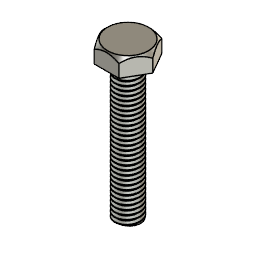
smartie_hopper (Autodesk Fusion 360 archive; units mm, degrees)
design "M6 32 mm Hex Bolt"
part number: 2026-04-25-09-17-42-437
Autodesk Fusion 360 part; units mm, degrees
sketch "Thread" plane through (0, 0, 0) normal (0, 0, 1) x (1, 0, 0)
  circle A0 centre (0, 0) radius 3
  dimension "d2" = 6
  constraint coincident A0.centre origin
  measures "d2" diameter of A0
extrude "Extrude1" add sketch "Thread" along normal blind 32
sketch "Head" plane through (0, 0, 32) normal (0, 0, 1) x (-1, 0, 0)
  circle A0 centre (0, 0) radius 3
  line L0 (2.8868, -5) -> (5.7735, 0)
  line L1 (5.7735, 0) -> (2.8868, 5)
  line L2 (2.8868, 5) -> (-2.8868, 5)
  line L3 (-2.8868, 5) -> (-5.7735, 0)
  line L4 (-5.7735, 0) -> (-2.8868, -5)
  line L5 (-2.8868, -5) -> (2.8868, -5)
  dimension "d10" = 10
  constraint coincident A0.centre origin
  measures "d10" distance of L2 L5
extrude "Extrude2" add sketch "Head" along normal blind 4 contours A0 | L0 L1 L2 L3 L4 L5
thread "Thread1" "ISO Metric profile 6.0 M6x1 M6x1 6g" major diameter 5.884 minor diameter 4.7435 pitch 1 angle 60 modelled right hand crest width 0.1444 on face at (2.9963, -0.1495, 21.3333) crest through (2.942, 0, -0.25)
sketch "Head fillet" plane through (0, 0, 0) normal (0, 1, 0) x (1, 0, 0)
  line L0 (2.8868, -32) -> (5.7735, -32)
  line L1 (5.7735, -32) -> (5.7735, -36)
  line L2 (5.7735, -36) -> (2.8868, -36)
  line L3 (2.8868, -36) -> (2.8868, -32)
  line L4 (-5.7735, -32) -> (-2.8868, -32)
  line L5 (-2.8868, -32) -> (-2.8868, -36)
  line L6 (-2.8868, -36) -> (-5.7735, -36)
  line L7 (-5.7735, -36) -> (-5.7735, -32)
  line L8 (-2.8868, -32) -> (2.8868, -32)
  line L9 (2.8868, -32) -> (2.8868, -36)
  line L10 (2.8868, -36) -> (-2.8868, -36)
  line L11 (-2.8868, -36) -> (-2.8868, -32)
  line L12 (5.7735, -36) -> (4.7735, -36)
  line L13 (5.7735, -36) -> (5.7735, -35)
  line L14 (4.7735, -36) -> (5.7735, -35)
  dimension "d14" = 1
  dimension "d15" = 1
  constraint coincident L1.end L2.start
  constraint perpendicular L1 L12
  constraint perpendicular L2 L13
  measures "d14" distance of L1.end L12.end
  measures "d15" distance of L1.end L13.end
revolve "Revolve1" cut sketch "Head fillet" angle 360 about axis through (0, 0, 1.75) along (0, 0, 1) contours L1 L2 L12 L13 L14
equation "diameter = 6 mm" comment "An M6 hex bolt has a diameter of 6 mm."
equation "d2 = diameter"
equation "thread_height = 32 mm" comment "The length of the M6 hex bolt (excluding the head)."
equation "d4 = thread_height"
equation "head_height = 4 mm" comment "An M6 hex bolt has a head thickness of 4 mm."
equation "width_across_flats = 10 mm" comment "An M6 hex bolt has a width across the flats of 10 mm."
equation "d10 = width_across_flats"
equation "d11 = head_height"
equation "chamfer_side_length = 1 mm" comment "Chamfer on the top of the hex bolt head."
equation "d14 = chamfer_side_length"
equation "d15 = chamfer_side_length"
named bodies: "M6 32 mm Hex Bolt"

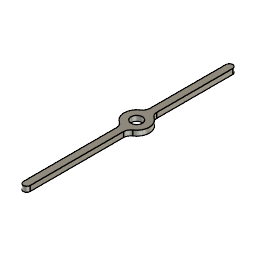
design "Mixer Arm"
part number: 2026-05-20-12-12-58-237
Autodesk Fusion 360 part; units mm, degrees
sketch "Mixer arm" plane through (0, 0, 0) normal (0, 0, 1) x (1, 0, 0)
  circle A0 centre (0, 0) radius 7.25
  circle A1 centre (0, 0) radius 3.25
  line L0 (-2, 55.25) -> (2, 55.25)
  line L1 (2, 55.25) -> (2, 3.25)
  line L2 (2, 3.25) -> (-2, 3.25)
  line L3 (-2, 3.25) -> (-2, 55.25)
  line L4 (-2, -3.25) -> (2, -3.25)
  line L5 (2, -3.25) -> (2, -65.25)
  line L6 (2, -65.25) -> (-2, -65.25)
  line L7 (-2, -65.25) -> (-2, -3.25)
  line L8 (-2, -7.25) -> (2, -7.25)
  line L9 (-2, 7.25) -> (2, 7.25)
  dimension "d3" = 6.5
  dimension "d5" = 14.5
  dimension "d6" = 2
  dimension "d7" = 2
  dimension "d8" = 2
  dimension "d9" = 2
  dimension "d14" = 58
  dimension "d15" = 48
  constraint coincident A0.centre A1.centre
  constraint concentric A0 A1
  constraint horizontal L0
  constraint vertical L1
  constraint horizontal L2
  constraint vertical L3
  constraint horizontal L4
  constraint vertical L5
  constraint horizontal L6
  constraint vertical L7
  constraint tangent A1 L2
  constraint tangent A1 L4
  constraint coincident L7 L8.start
  constraint coincident L5 L8.end
  constraint perpendicular L5 L8
  constraint tangent A0 L8
  constraint coincident L1 L9.end
  constraint perpendicular L1 L9
  constraint tangent A0 L9
  measures "d3" diameter of A1
  measures "d5" diameter of A0
  measures "d6" distance of A0.centre L1
  measures "d7" distance of A0.centre L3
  measures "d8" distance of A0.centre L7
  measures "d9" distance of A0.centre L5
  measures "d14" distance of L6 L8
  measures "d15" distance of L0 L9
extrude "Extrude1" add sketch "Mixer arm" along normal blind 3 contours A0 A1 L1 L2 L4 L5 | A0 L1 L2 L3 | A0 L1 L9 | A0 L5 L8 | A0 L4 L5 L7 | A0 L3 L9 | L0 L1 L3 L9 | A0 L7 L8 | L5 L6 L7 L8 | A0 A1 L2 L3 L4 L7
fillet "Fillet1" radius 4 4 edges at (2, -6.9687, 1.5) (2, 6.9687, 1.5) (-2, 6.9687, 1.5) (-2, -6.9687, 1.5)
fillet "Fillet2" radius 2 4 edges at (2, 55.25, 1.5) (-2, 55.25, 1.5) (-2, -65.25, 1.5) (2, -65.25, 1.5)
equation "stainless_steel_thickness = 3 mm" comment "The thickness of the 316 stainless steel sheets to laser cut."
equation "hole_diameter = 6.5 mm"
equation "d3 = hole_diameter"
equation "arm_thickness = 4 mm"
equation "d5 = hole_diameter + 2 * arm_thickness"
equation "d6 = arm_thickness / 2"
equation "d7 = arm_thickness / 2"
equation "d8 = arm_thickness / 2"
equation "d9 = arm_thickness / 2"
equation "d10 = stainless_steel_thickness"
equation "arm_length_front = 58 mm"
equation "arm_length_back = 48 mm"
equation "d14 = arm_length_front"
equation "d15 = arm_length_back"
equation "d17 = arm_thickness"
equation "d19 = arm_thickness / 2"
named bodies: "Mixer arm"

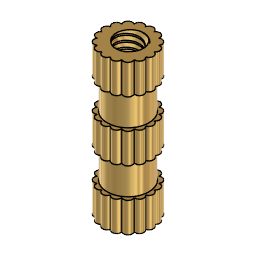
design "M2 10 mm Threaded Brass Insert"
part number: 2026-06-20-09-24-02-047
Autodesk Fusion 360 part; units mm, degrees
sketch "Brass thread outline" plane through (0, 0, 0) normal (0, 0, 1) x (1, 0, 0)
  circle A0 centre (0, 0) radius 1.4
  dimension "d4" = 2.8
  constraint coincident A0.centre origin
  measures "d4" diameter of A0
extrude "Extrude1" add sketch "Brass thread outline" along normal blind 10
sketch "Ridges" plane through (0, 0, 10) normal (0, 0, 1) x (-1, 0, 0)
  circle A0 centre (0, 0) radius 1.4
  circle A1 centre (0, 0) radius 1.7
  circle A2 centre (-0.0001, -1.4) radius 0.3
  circle A3 centre (0.5357, -1.2935) radius 0.3
  circle A4 centre (0.9899, -0.99) radius 0.3
  circle A5 centre (1.2934, -0.5358) radius 0.3
  circle A6 centre (1.4, -0.0001) radius 0.3
  circle A7 centre (1.2935, 0.5357) radius 0.3
  circle A8 centre (0.99, 0.9899) radius 0.3
  circle A9 centre (0.5358, 1.2934) radius 0.3
  circle A10 centre (0.0001, 1.4) radius 0.3
  circle A11 centre (-0.5357, 1.2935) radius 0.3
  circle A12 centre (-0.9899, 0.99) radius 0.3
  circle A13 centre (-1.2934, 0.5358) radius 0.3
  circle A14 centre (-1.4, 0.0001) radius 0.3
  circle A15 centre (-1.2935, -0.5357) radius 0.3
  circle A16 centre (-0.99, -0.9899) radius 0.3
  circle A17 centre (-0.5358, -1.2934) radius 0.3
  dimension "d8" = 3.4
  dimension "d29" = 0.0001
  dimension "d31" = 360
  constraint coincident A0.centre A1.centre
  constraint coincident A0 A2.centre
  constraint tangent A1 A2
  measures "d8" diameter of A1
  measures "d29" horizontal distance of A0.centre A2.centre
extrude "Extrude2" add sketch "Ridges" against normal blind 2 contours A0 A5 A6 A7 | A0 A5 A6 A7 | A0 A6 A7 | A0 A6 A7 | A0 A5 A6 | A0 A5 A6 | A0 A6 A7 A8 | A0 A6 A7 A8 | A2 A3 A4 A5 A6 A7 A8 A9 A10 A11 A12 A13 A14 A15 A16 A17 | A0 A4 A5 A6 | A0 A4 A5 A6 | A0 A7 A8 | A0 A7 A8 | A0 A7 A8 A9 | A0 A4 A5 | A0 A4 A5 | A0 A3 A4 A5 | A0 A7 A8 A9 | A0 A8 A9 A10 | A0 A8 A9 | A0 A3 A4 A5 | A0 A2 A3 A4 | A0 A3 A4 | A0 A8 A9 | A0 A8 A9 A10 | A0 A9 A10 A11 | A0 A9 A10 | A0 A3 A4 | A0 A2 A3 A17 | A0 A2 A3 | A0 A2 A3 A4 | A0 A9 A10 | A0 A9 A10 A11 | A0 A10 A11 A12 | A0 A10 A11 | A0 A2 A3 | A0 A2 A17 | A0 A2 A16 A17 | A0 A2 A3 A17 | A0 A10 A11 | A0 A10 A11 A12 | A0 A11 A12 A13 | A0 A11 A12 | A0 A2 A16 A17 | A0 A2 A17 | A0 A15 A16 A17 | A0 A16 A17 | A0 A11 A12 | A0 A11 A12 A13 | A0 A16 A17 | A0 A15 A16 A17 | A0 A12 A13 | A0 A12 A13 | A0 A12 A13 A14 | A0 A14 A15 A16 | A0 A15 A16 | A0 A15 A16 | A0 A12 A13 A14 | A0 A14 A15 A16 | A0 A13 A14 | A0 A13 A14 | A0 A13 A14 A15 | A0 A13 A14 A15 | A0 A14 A15 | A0 A14 A15
pattern_linear "R-Pattern1" count 3 spacing 4 along (0, 0, -1) of "Extrude2"
sketch "Thread hole" plane through (0, 0, 10) normal (0, 0, 1) x (-1, 0, 0)
  circle A0 centre (0, 0) radius 1
  arc A1 (0.292, -1.4685) -> (0.8317, -1.2449) centre (0.5357, -1.2935) ccw
  arc A2 (0.8317, -1.2449) -> (1.2448, -0.8319) centre (0.9899, -0.99) ccw
  arc A3 (1.2448, -0.8319) -> (1.4684, -0.2922) centre (1.2934, -0.5358) ccw
  arc A4 (1.4684, -0.2922) -> (1.4685, 0.292) centre (1.4, -0.0001) ccw
  arc A5 (1.4685, 0.292) -> (1.2449, 0.8317) centre (1.2935, 0.5357) ccw
  arc A6 (1.2449, 0.8317) -> (0.8319, 1.2448) centre (0.99, 0.9899) ccw
  arc A7 (0.8319, 1.2448) -> (0.2922, 1.4684) centre (0.5358, 1.2934) ccw
  arc A8 (0.2922, 1.4684) -> (-0.292, 1.4685) centre (0.0001, 1.4) ccw
  arc A9 (-0.292, 1.4685) -> (-0.8317, 1.2449) centre (-0.5357, 1.2935) ccw
  arc A10 (-0.8317, 1.2449) -> (-1.2448, 0.8319) centre (-0.9899, 0.99) ccw
  arc A11 (-1.2448, 0.8319) -> (-1.4684, 0.2922) centre (-1.2934, 0.5358) ccw
  arc A12 (-1.4684, 0.2922) -> (-1.4685, -0.292) centre (-1.4, 0.0001) ccw
  arc A13 (-1.4685, -0.292) -> (-1.2449, -0.8317) centre (-1.2935, -0.5357) ccw
  arc A14 (-1.2449, -0.8317) -> (-0.8319, -1.2448) centre (-0.99, -0.9899) ccw
  arc A15 (-0.8319, -1.2448) -> (-0.2922, -1.4684) centre (-0.5358, -1.2934) ccw
  arc A16 (-0.2922, -1.4684) -> (0.292, -1.4685) centre (-0.0001, -1.4) ccw
  dimension "d11" = 2
  constraint coincident A0.centre origin
  measures "d11" diameter of A0
extrude "Extrude3" cut sketch "Thread hole" against normal blind 10 contours A0
thread "Thread1" "ISO Metric profile 2.0 M2x0.4 M2x0.4 6H" major diameter 2.074 minor diameter 1.623 pitch 0.4 angle 60 modelled right hand crest width 0.1065 on face at (-0.9988, 0.0498, 3.3333) crest through (-0.8115, 0, 9.9)
equation "outer_diameter = 2.8 mm" comment "The outer diameter of the non-ridged parts."
equation "hole_diameter = 2 mm" comment "The thread diameter of the brass insert. 2 mm for this M2 insert."
equation "height = 10 mm" comment "The height of the brass thread insert. 10 mm for this model."
equation "d4 = outer_diameter"
equation "d5 = height"
equation "ridge_diameter = 3.4 mm" comment "The outer diameter of the ridged parts."
equation "d8 = ridge_diameter"
equation "d9 = -ridge_height"
equation "d11 = hole_diameter"
equation "d12 = -height"
equation "number_of_ridges = 3" comment "The number of ridges to have along the outside."
equation "d23 = number_of_ridges"
equation "d25 = -ridge_pattern_length"
equation "ridge_pattern_length = height - ridge_height" comment "The distance to use for the rectangular pattern that repeats the ridges."
equation "ridge_height = 2 mm" comment "The height of the individual ridges."
named bodies: "M2 10 mm Threaded Brass Insert"

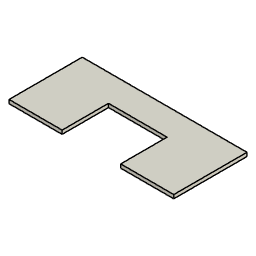
design "Colour Detection Mechanism Top Panel"
part number: 2025-05-13-09-48-31-121
Autodesk Fusion 360 part; units mm, degrees
sketch "Sorting Mechanism Top Panel" plane through (0, 0, 0) normal (0, 0, 1) x (1, 0, 0)
  line L0 (0, 0) -> (270, 0)
  line L1 (270, 0) -> (270, 120)
  line L2 (270, 120) -> (0, 120)
  line L3 (0, 120) -> (0, 0)
  dimension "d1" = 270
  dimension "d2" = 120
  constraint horizontal L0
  constraint vertical L1
  constraint horizontal L2
  constraint vertical L3
  constraint coincident L0.start L3.end
  measures "d1" distance of L0.start L0.end
  measures "d2" distance of L0.end L1.end
extrude "Extrude1" add sketch "Sorting Mechanism Top Panel" along normal blind 6
sketch "Smartie Hopper Hole" plane through (0, 0, 6) normal (0, 0, 1) x (-1, 0, 0)
  line L0 (0, -120) -> (0, 0)
  line L1 (0, 0) -> (-270, 0)
  line L2 (-270, 0) -> (-270, -120)
  line L3 (-270, -120) -> (0, -120)
  line L4 (-87, -76) -> (-183, -76)
  line L5 (-183, -76) -> (-183, 0)
  line L6 (-183, 0) -> (-87, 0)
  line L7 (-87, 0) -> (-87, -76)
  dimension "d7" = 96
  dimension "d9" = 76
  dimension "d10" = 87
  dimension "d11" = 87
  constraint horizontal L4
  constraint vertical L5
  constraint horizontal L6
  constraint vertical L7
  constraint collinear L1 L6
  measures "d7" distance of L4.start L4.end
  measures "d9" distance of L4.end L5.end
  measures "d10" distance of L0 L7
  measures "d11" distance of L2 L5
extrude "Extrude2" cut sketch "Smartie Hopper Hole" against normal blind 6 contours L1 L4 L5 L6 L7
equation "d3 = MDF_thickness"
equation "acrylic_thickness = 3 mm" comment "Thickness of the clear acrylic panels"
equation "MDF_thickness = 6 mm" comment "Thickness of the MDF panels"
equation "d7 = smarties_hopper_width + 2 * acrylic_thickness"
equation "smarties_hopper_width = 90 mm" comment "Width of the Smarties hopper"
equation "d9 = smarties_hopper_depth + 2 * acrylic_thickness"
equation "d10 = ( 270 mm - ( smarties_hopper_width + 2 * acrylic_thickness ) ) / 2"
equation "d14 = -MDF_thickness"
equation "smarties_hopper_depth = 70 mm" comment "Depth of the Smarties hopper"
named bodies: "Sorting Mechanism Top Panel"

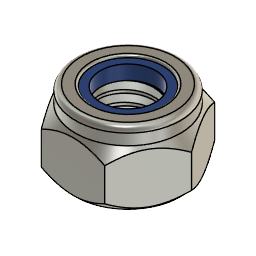
design "M6 Nylock Hex Nut"
part number: 2026-04-25-09-47-30-495
Autodesk Fusion 360 part; units mm, degrees
sketch "Hex Nut Shape" plane through (0, 0, 0) normal (0, 0, 1) x (1, 0, 0)
  line L0 (-2.8868, 5) -> (-5.7735, 0)
  line L1 (-5.7735, 0) -> (-2.8868, -5)
  line L2 (-2.8868, -5) -> (2.8868, -5)
  line L3 (2.8868, -5) -> (5.7735, 0)
  line L4 (5.7735, 0) -> (2.8868, 5)
  line L5 (2.8868, 5) -> (-2.8868, 5)
  dimension "d3" = 10
  measures "d3" distance of L2 L5
extrude "Extrude1" add sketch "Hex Nut Shape" along normal blind 5 makes body 1
sketch "Chamfer Outline" plane through (0, 0, 0) normal (0, 1, 0) x (1, 0, 0)
  line L0 (2.8868, 0) -> (5.7735, 0)
  line L1 (5.7735, 0) -> (5.7735, -5)
  line L2 (5.7735, -5) -> (2.8868, -5)
  line L3 (2.8868, -5) -> (2.8868, 0)
  line L4 (-2.8868, 0) -> (2.8868, 0)
  line L5 (2.8868, 0) -> (2.8868, -5)
  line L6 (2.8868, -5) -> (-2.8868, -5)
  line L7 (-2.8868, -5) -> (-2.8868, 0)
  line L8 (-5.7735, 0) -> (-2.8868, 0)
  line L9 (-2.8868, 0) -> (-2.8868, -5)
  line L10 (-2.8868, -5) -> (-5.7735, -5)
  line L11 (-5.7735, -5) -> (-5.7735, 0)
  line L12 (5.7735, -5) -> (4.7735, -5)
  line L13 (5.7735, -5) -> (5.7735, -4)
  line L14 (5.7735, 0) -> (5.7735, -1)
  line L15 (5.7735, 0) -> (4.7735, 0)
  line L16 (4.7735, -5) -> (5.7735, -4)
  line L17 (5.7735, -1) -> (4.7735, 0)
  dimension "d11" = 1
  dimension "d12" = 1
  dimension "d13" = 1
  dimension "d14" = 1
  constraint coincident L1.end L2.start
  constraint perpendicular L1 L12
  constraint coincident L1 L13.end
  constraint coincident L0.end L1.start
  constraint perpendicular L2 L14
  constraint perpendicular L14 L15
  measures "d11" distance of L1.end L12.end
  measures "d12" distance of L1.end L13.end
  measures "d13" distance of L0.end L14.end
  measures "d14" distance of L0.end L15.end
revolve "Revolve1" cut sketch "Chamfer Outline" angle 360 about axis through (0, 0, 1.75) along (0, 0, 1) contours L0 L1 L14 L15 L17 | L1 L2 L12 L13 L16 bodies 1
hole "Hole1" at (0, 0, 5) direction (0, 0, -1) diameter 6 end through all bodies 1
chamfer "Chamfer1" distance 0.25 angle 45 1 edges at (-2.797, -1.0848, 0) on bodies 1
thread "Thread1" "ISO Metric profile 6.0 M6x1 M6x1 6H" major diameter 6.147 minor diameter 5.035 pitch 1 angle 60 modelled right hand crest width 0.2748 on face at (0.2987, -2.9851, 3.4167) crest through (2.5175, 0, 4.75) on bodies 1
sketch "Nylock Outline" plane through (0, 0, 5) normal (0, 0, 1) x (-1, 0, 0)
  spline S0 degree 3 poles (0.7938, 2.9692) (1.1619, 2.8346) (1.5007, 2.6305) (2.069, 2.1114) (2.2965, 1.8052) (2.6132, 1.1343) (2.704, 0.7783) (2.7408, 0.0652) (2.6916, -0.2847) (2.5067, -0.8107) (2.4149, -0.9977) (2.1912, -1.3413) (2.061, -1.4974) (1.9135, -1.636) knots 0 0 0 0 0.117588 0.117588 0.231087 0.231087 0.340498 0.340498 0.445817 0.445817 0.508297 0.508297 0.569249 0.569249 0.569249 0.569249
  arc A0 (-1.9135, -1.636) -> (1.9135, -1.636) centre (0, 0) ccw
  spline S1 degree 3 poles (-1.9135, -1.636) (-2.1558, -1.4082) (-2.3504, -1.1345) (-2.6319, -0.5162) (-2.7113, -0.1755) (-2.7381, 0.5311) (-2.68, 0.8904) (-2.4271, 1.5805) (-2.2298, 1.9028) (-1.817, 2.3542) (-1.6364, 2.5092) (-1.2382, 2.776) (-1.0214, 2.886) (-0.7938, 2.9692) knots 0 0 0 0 0.09977 0.09977 0.203618 0.203618 0.311544 0.311544 0.423544 0.423544 0.494428 0.494428 0.566847 0.566847 0.566847 0.566847
  arc A1 (0.7938, 2.9692) -> (-0.7938, 2.9692) centre (0, 0) ccw
  circle A2 centre (0, 0) radius 4.7735
  circle A3 centre (0, 0) radius 2.5
  circle A4 centre (0, 0) radius 3.2
  dimension "d23" = 5
  dimension "d24" = 0.7
  constraint concentric A0 A3
  constraint concentric A0 A4
  measures "d23" diameter of A3
  measures "d24" distance of A3 A4
extrude "Extrude2" add sketch "Nylock Outline" along normal blind 1.3 separate body contours S0 A0 S1 A1 | A4 makes body 2
extrude "Extrude3" add sketch "Nylock Outline" along normal blind 1.5 contours A2 bodies 1
fillet "Fillet2" radius 0.5 1 edges at (4.4505, 1.7262, 6.5) on bodies 1
fillet "Fillet3" radius 0.2 1 edges at (2.9834, -1.1572, 6.5) on bodies 1
equation "width_across_flats = 10 mm" comment "An M6 hex nut has a widths across the flats of 10 mm."
equation "thickness = 5 mm" comment "An M6 hex nut has a thickness of 5 mm."
equation "d3 = width_across_flats"
equation "d4 = thickness"
equation "chamfer_side_length = 1 mm" comment "Chamfer on the outside top and bottom of the hex nut."
equation "d11 = chamfer_side_length"
equation "d12 = chamfer_side_length"
equation "d13 = chamfer_side_length"
equation "d14 = chamfer_side_length"
equation "d16 = hole_diameter"
equation "hole_diameter = 6 mm" comment "An M6 hex nut has a hole diameter of 6 mm."
equation "hole_chamfer = 0.25 mm" comment "Chamfer on the inside of the hex nut thread hole."
equation "d20 = hole_chamfer"
equation "d23 = hole_diameter - 1 mm"
equation "d24 = nylon_thickness"
equation "nylon_thickness = 0.7 mm" comment "The thickness of the nylon insert for the Nylock hex nut."
equation "top_height = 1.5 mm" comment "The height of the top portion containing the nylon insert."
equation "d27 = nylon_height"
equation "d29 = top_height"
equation "d35 = top_outside_fillet_radius"
equation "top_outside_fillet_radius = 0.5 mm" comment "The radius of the fillet on the outside of the top portion containing the nylon insert."
equation "nylon_height = top_height - top_inside_fillet_radius" comment "The height of the nylon insert for the Nylock hex nut."
equation "top_inside_fillet_radius = 0.2 mm" comment "The radius of the fillet on the inside of the top portion containing the nylon insert."
equation "d40 = top_inside_fillet_radius"
named bodies: "M6 Hex Nut", "Nylon Insert"

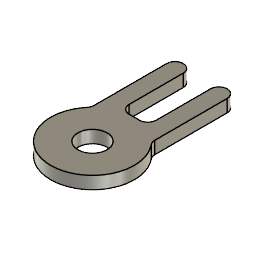
design "Smartie Hopper Servo Arm"
part number: 2026-05-20-12-12-58-237
Autodesk Fusion 360 part; units mm, degrees
sketch "Smartie Hopper servo arm" plane through (0, 0, 0) normal (0, 0, 1) x (1, 0, 0)
  circle A0 centre (0, 0) radius 10
  circle A1 centre (0, 0) radius 3.5
  line L0 (-3.25, 25) -> (-3.25, 10)
  line L1 (3.25, 25) -> (3.25, 10)
  line L2 (-7.25, 25) -> (-7.25, 6.8875)
  line L3 (7.25, 25) -> (7.25, 6.8875)
  line L4 (-3.25, 10) -> (3.25, 10)
  line L5 (-7.25, 25) -> (-3.25, 25)
  line L6 (3.25, 25) -> (7.25, 25)
  circle A2 centre (-5.25, 25) radius 2
  circle A3 centre (5.25, 25) radius 2
  dimension "d3" = 7
  dimension "d5" = 20
  dimension "d28" = 3.25
  dimension "d29" = 3.25
  dimension "d34" = 4
  dimension "d35" = 4
  dimension "d36" = 15
  dimension "d37" = 15
  dimension "d38" = 4
  dimension "d39" = 4
  constraint coincident A0.centre A1.centre
  constraint concentric A0 A1
  constraint vertical L0
  constraint coincident A0 L2.end
  constraint vertical L2
  constraint coincident A0 L3.end
  constraint parallel L2 L3
  constraint perpendicular L1 L4
  constraint tangent A0 L4
  constraint perpendicular L0 L5
  constraint coincident L1 L6.start
  constraint perpendicular L1 L6
  constraint midpoint L5 A2.centre
  constraint midpoint L6 A3.centre
  constraint horizontal L4
  measures "d3" diameter of A1
  measures "d5" diameter of A0
  measures "d28" horizontal distance of A0.centre L0.end
  measures "d29" horizontal distance of A0.centre L1.end
  measures "d34" diameter of A2
  measures "d35" diameter of A3
  measures "d36" distance of L4 A3.centre
  measures "d37" distance of L4 A2.centre
  measures "d38" distance of L0 L2
  measures "d39" distance of L1 L3
extrude "Extrude1" add sketch "Smartie Hopper servo arm" along normal blind 3
fillet "Fillet4" radius 2 2 edges at (3.25, 10, 1.5) (-3.25, 10, 1.5)
fillet "Fillet3" radius 2 2 edges at (7.25, 6.8875, 1.5) (-7.25, 6.8875, 1.5)
equation "stainless_steel_thickness = 3 mm" comment "The thickness of the 316 stainless steel sheets to laser cut."
equation "arm_thickness = 4 mm"
equation "d10 = stainless_steel_thickness"
equation "groove_diameter = 6.5 mm"
equation "groove_length = 17 mm"
equation "d28 = groove_diameter / 2"
equation "d29 = groove_diameter / 2"
equation "d34 = arm_thickness"
equation "d35 = arm_thickness"
equation "d36 = groove_length - ( arm_thickness / 2 )"
equation "d37 = groove_length - ( arm_thickness / 2 )"
equation "d38 = arm_thickness"
equation "d39 = arm_thickness"
equation "d19 = arm_thickness / 2"
named bodies: "Smartie Hopper servo arm"

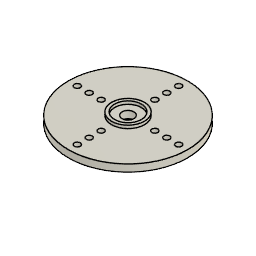
design "Savöx SH 0255 MG Micro Servo Horn"
description: Spur Gear; Module: 0.217; Num Teeth: 21; Pressure Angle: 20.0; Backlash: 0.00 mm
part number: 2026-07-12-11-53-48-100
Autodesk Fusion 360 part; units mm, degrees
sketch "Horn body" plane through (0, 0, 0) normal (0, 0, 1) x (1, 0, 0)
  circle A0 centre (0, 0) radius 10
  dimension "d1" = 20
  constraint coincident A0.centre origin
  measures "d1" diameter of A0
extrude "Extrude1" add sketch "Horn body" along normal blind 1.2 makes body 1
sketch "Connector" plane through (0, 0, 0) normal (0, 0, -1) x (1, 0, 0)
  circle A0 centre (0, 0) radius 10
  circle A1 centre (0, 0) radius 3.5
  dimension "d5" = 7
  constraint coincident A0.centre A1.centre
  measures "d5" diameter of A1
extrude "Extrude2" add sketch "Connector" along normal blind 3 contours A1 bodies 1
sketch "Screw hole" plane through (0, 0, 1.2) normal (0, 0, 1) x (-1, 0, 0)
  circle A0 centre (0, 0) radius 10
  circle A1 centre (0, 0) radius 2.75
  circle A2 centre (0, 0) radius 2.25
  circle A3 centre (0, 0) radius 1
  dimension "d8" = 5.5
  dimension "d9" = 4.5
  dimension "d10" = 2
  constraint coincident A0.centre A1.centre
  constraint concentric A2 A3
  measures "d8" diameter of A1
  measures "d9" diameter of A2
  measures "d10" diameter of A3
extrude "Extrude3" add sketch "Screw hole" along normal blind 0.5 contours A1 bodies 1
extrude "Extrude4" cut sketch "Screw hole" against normal blind 1.2 contours A3 bodies 1
sketch "Top small holes" plane through (0, 0, 1.2) normal (0, 0, 1) x (-1, 0, 0)
  circle A0 centre (0, 0) radius 10
  circle A1 centre (0, 0) radius 2.75
  circle A2 centre (0, -8.5) radius 0.5
  circle A3 centre (0, -6.5) radius 0.5
  circle A4 centre (0, -4.5) radius 0.5
  dimension "d15" = 1
  dimension "d16" = 1
  dimension "d17" = 1
  dimension "d19" = 8.5
  dimension "d20" = 6.5
  dimension "d21" = 4.5
  measures "d15" diameter of A2
  measures "d16" diameter of A3
  measures "d17" diameter of A4
  measures "d19" distance of A0.centre A2.centre
  measures "d20" distance of A0.centre A3.centre
  measures "d21" distance of A0.centre A4.centre
extrude "Extrude5" cut sketch "Top small holes" against normal blind 1.2 contours A2 | A3 | A4 bodies 1
pattern_circular "C-Pattern1" count 4 over 360 about axis through (0, 0, 1.75) along (0, 0, 1) of "Extrude5"
sketch "Base Circle" plane through (0, 0, 0) normal (0, 0, 1) x (1, 0, 0) in component "Savöx SH 0255 MG Micro Servo Gear"
  circle A0 centre (0, 0) radius 2.0274
extrude "Extrude1'" add sketch "Base Circle" along normal blind 3 separate body makes body 2 in component "Savöx SH 0255 MG Micro Servo Gear"
sketch "Gear Tooth" plane through (0, 0, 0) normal (0, 0, 1) x (1, 0, 0) in component "Savöx SH 0255 MG Micro Servo Gear"
  spline S0 degree 5 poles (2.1325, -0.1918) (2.1335, -0.1919) (2.1355, -0.1921) (2.1386, -0.1922) (2.1427, -0.1923) (2.1478, -0.1921) (2.1529, -0.1919) (2.1581, -0.1915) (2.1632, -0.191) (2.1683, -0.1906) (2.1735, -0.1901) (2.1787, -0.1895) (2.1838, -0.1889) (2.189, -0.1882) (2.1941, -0.1875) (2.1993, -0.1867) (2.2045, -0.1858) (2.2097, -0.1849) (2.2148, -0.1839) (2.22, -0.1829) (2.2252, -0.1818) (2.2304, -0.1807) (2.2356, -0.1796) (2.2407, -0.1784) (2.2459, -0.1772) (2.2511, -0.1759) (2.2563, -0.1746) (2.2615, -0.1732) (2.2667, -0.1718) (2.2719, -0.1703) (2.2771, -0.1689) (2.2823, -0.1674) (2.2875, -0.1658) (2.2927, -0.1642) (2.2979, -0.1626) (2.3031, -0.1609) (2.3083, -0.1592) (2.3134, -0.1575) (2.3186, -0.1557) (2.3238, -0.1539) (2.329, -0.152) (2.3342, -0.1502) (2.3394, -0.1482) (2.3446, -0.1463) (2.3498, -0.1443) (2.355, -0.1423) (2.3602, -0.1403) (2.3654, -0.1382) (2.3705, -0.1361) (2.3757, -0.1339) (2.3809, -0.1317) (2.3861, -0.1295) (2.3913, -0.1273) (2.3964, -0.125) (2.4016, -0.1227) (2.4068, -0.1204) (2.412, -0.118) (2.4171, -0.1156) (2.4223, -0.1132) (2.4275, -0.1107) (2.4326, -0.1082) (2.4378, -0.1057) (2.4429, -0.1032) (2.4481, -0.1006) (2.4532, -0.098) (2.4584, -0.0953) (2.4635, -0.0927) (2.4687, -0.09) (2.4738, -0.0872) (2.479, -0.0845) (2.4841, -0.0817) (2.4882, -0.0794) (2.4913, -0.0777) (2.4933, -0.0766) (2.4943, -0.076) knots 0 0 0 0 0 0 0.01428571 0.02857143 0.04285714 0.05714286 0.07142857 0.08571429 0.1 0.11428571 0.12857143 0.14285714 0.15714286 0.17142857 0.18571429 0.2 0.21428571 0.22857143 0.24285714 0.25714286 0.27142857 0.28571429 0.3 0.31428571 0.32857143 0.34285714 0.35714286 0.37142857 0.38571429 0.4 0.41428571 0.42857143 0.44285714 0.45714286 0.47142857 0.48571429 0.5 0.51428571 0.52857143 0.54285714 0.55714286 0.57142857 0.58571429 0.6 0.61428571 0.62857143 0.64285714 0.65714286 0.67142857 0.68571429 0.7 0.71428571 0.72857143 0.74285714 0.75714286 0.77142857 0.78571429 0.8 0.81428571 0.82857143 0.84285714 0.85714286 0.87142857 0.88571429 0.9 0.91428571 0.92857143 0.94285714 0.95714286 0.97142857 0.98571429 1 1 1 1 1 1
  spline S1 degree 5 poles (2.1325, 0.1918) (2.1335, 0.1919) (2.1355, 0.1921) (2.1386, 0.1922) (2.1427, 0.1923) (2.1478, 0.1921) (2.1529, 0.1919) (2.1581, 0.1915) (2.1632, 0.191) (2.1683, 0.1906) (2.1735, 0.1901) (2.1787, 0.1895) (2.1838, 0.1889) (2.189, 0.1882) (2.1941, 0.1875) (2.1993, 0.1867) (2.2045, 0.1858) (2.2097, 0.1849) (2.2148, 0.1839) (2.22, 0.1829) (2.2252, 0.1818) (2.2304, 0.1807) (2.2356, 0.1796) (2.2407, 0.1784) (2.2459, 0.1772) (2.2511, 0.1759) (2.2563, 0.1746) (2.2615, 0.1732) (2.2667, 0.1718) (2.2719, 0.1703) (2.2771, 0.1689) (2.2823, 0.1674) (2.2875, 0.1658) (2.2927, 0.1642) (2.2979, 0.1626) (2.3031, 0.1609) (2.3083, 0.1592) (2.3134, 0.1575) (2.3186, 0.1557) (2.3238, 0.1539) (2.329, 0.152) (2.3342, 0.1502) (2.3394, 0.1482) (2.3446, 0.1463) (2.3498, 0.1443) (2.355, 0.1423) (2.3602, 0.1403) (2.3654, 0.1382) (2.3705, 0.1361) (2.3757, 0.1339) (2.3809, 0.1317) (2.3861, 0.1295) (2.3913, 0.1273) (2.3964, 0.125) (2.4016, 0.1227) (2.4068, 0.1204) (2.412, 0.118) (2.4171, 0.1156) (2.4223, 0.1132) (2.4275, 0.1107) (2.4326, 0.1082) (2.4378, 0.1057) (2.4429, 0.1032) (2.4481, 0.1006) (2.4532, 0.098) (2.4584, 0.0953) (2.4635, 0.0927) (2.4687, 0.09) (2.4738, 0.0872) (2.479, 0.0845) (2.4841, 0.0817) (2.4882, 0.0794) (2.4913, 0.0777) (2.4933, 0.0766) (2.4943, 0.076) knots 0 0 0 0 0 0 0.01428571 0.02857143 0.04285714 0.05714286 0.07142857 0.08571429 0.1 0.11428571 0.12857143 0.14285714 0.15714286 0.17142857 0.18571429 0.2 0.21428571 0.22857143 0.24285714 0.25714286 0.27142857 0.28571429 0.3 0.31428571 0.32857143 0.34285714 0.35714286 0.37142857 0.38571429 0.4 0.41428571 0.42857143 0.44285714 0.45714286 0.47142857 0.48571429 0.5 0.51428571 0.52857143 0.54285714 0.55714286 0.57142857 0.58571429 0.6 0.61428571 0.62857143 0.64285714 0.65714286 0.67142857 0.68571429 0.7 0.71428571 0.72857143 0.74285714 0.75714286 0.77142857 0.78571429 0.8 0.81428571 0.82857143 0.84285714 0.85714286 0.87142857 0.88571429 0.9 0.91428571 0.92857143 0.94285714 0.95714286 0.97142857 0.98571429 1 1 1 1 1 1
  arc A0 (2.4943, -0.076) -> (2.4943, 0.076) centre (0, 0) ccw
  line L0 (2.0093, -0.1807) -> (2.1325, -0.1918)
  line L1 (2.0093, 0.1807) -> (2.1325, 0.1918)
  line L2 (2.0093, -0.1807) -> (2.0093, 0.1807)
  point P0 (2.1579, -0.1915)
  point P1 (2.1836, -0.1889)
  point P2 (2.2093, -0.1849)
  point P3 (2.2351, -0.1797)
  point P4 (2.261, -0.1733)
  point P5 (2.287, -0.1659)
  point P6 (2.3129, -0.1576)
  point P7 (2.3389, -0.1484)
  point P8 (2.3649, -0.1384)
  point P9 (2.3908, -0.1275)
  point P10 (2.4168, -0.1158)
  point P11 (2.4427, -0.1033)
  point P12 (2.4685, -0.09)
  point P13 (2.1579, 0.1915)
  point P14 (2.1836, 0.1889)
  point P15 (2.2093, 0.1849)
  point P16 (2.2351, 0.1797)
  point P17 (2.261, 0.1733)
  point P18 (2.287, 0.1659)
  point P19 (2.3129, 0.1576)
  point P20 (2.3389, 0.1484)
  point P21 (2.3649, 0.1384)
  point P22 (2.3908, 0.1275)
  point P23 (2.4168, 0.1158)
  point P24 (2.4427, 0.1033)
  point P25 (2.4685, 0.09)
extrude "Extrude2'" add sketch "Gear Tooth" along normal blind 3 bodies 2 in component "Savöx SH 0255 MG Micro Servo Gear"
fillet "Fillet1" radius 0.1 2 edges at (2.0193, -0.1816, 1.5) (2.0193, 0.1816, 1.5) on bodies 2 in component "Savöx SH 0255 MG Micro Servo Gear"
pattern_circular "C-Pattern1'" count 21 over 360 about axis through (0, 0, 0) along (0, 0, 1) of "Extrude2'", "Fillet1" in component "Savöx SH 0255 MG Micro Servo Gear"
sketch "Diametrial Pitch Circle" plane through (0, 0, 0) normal (0, 0, 1) x (1, 0, 0) in component "Savöx SH 0255 MG Micro Servo Gear"
  circle A0 centre (0, 0) radius 2.2785 construction
move_body "Move1" bodies 2 to x (1, 0, 0) y (0, 1, 0) z (0, 0, 1) at (0, 0, -3) in component "Savöx SH 0255 MG Micro Servo Gear"
combine "Combine1" operation cut target body 1 tool bodies 2 keep tools
component "Savöx SH 0255 MG Micro Servo Gear" placed x (1, 0, 0) y (0, 1, 0) z (0, 0, 1) at (0, 0, 0)
named bodies: "Savöx SH 0255 MG Micro Servo Horn", "Savöx SH 0255 MG Micro Servo Gear"

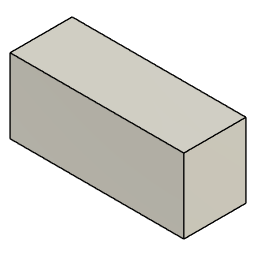
design "Colour Detection Mechanism Top Panel Placeholder"
part number: 2025-05-14-09-44-42-407
Autodesk Fusion 360 part; units mm, degrees
sketch "Sorting Mechanism Top Panel Placeholder" plane through (0, 0, 0) normal (0, 0, 1) x (1, 0, 0)
  line L0 (0, 0) -> (28, 0)
  line L1 (28, 0) -> (28, 10)
  line L2 (28, 10) -> (0, 10)
  line L3 (0, 10) -> (0, 0)
  dimension "d1" = 10
  dimension "d2" = 28
  constraint horizontal L0
  constraint vertical L1
  constraint horizontal L2
  constraint vertical L3
  constraint coincident L0.start L3.end
  measures "d1" distance of L0.end L1.end
  measures "d2" distance of L0.start L0.end
extrude "Extrude1" add sketch "Sorting Mechanism Top Panel Placeholder" along normal blind 12
named bodies: "Sorting Mechanism Top Panel Placeholder"

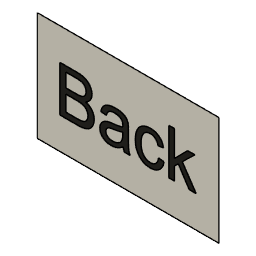
design "Back Label"
part number: 2025-04-13-10-14-33-970
Autodesk Fusion 360 part; units mm, degrees
sketch "Sticker" plane through (0, 0, 0) normal (0, 1, 0) x (1, 0, 0)
  line L0 (0, 0) -> (20, 0)
  line L1 (20, 0) -> (20, -12)
  line L2 (20, -12) -> (0, -12)
  line L3 (0, -12) -> (0, 0)
  dimension "d1" = 12
  dimension "d2" = 20
  constraint horizontal L0
  constraint vertical L1
  constraint horizontal L2
  constraint vertical L3
  constraint coincident L0.start L3.end
  measures "d1" distance of L0.end L1.end
  measures "d2" distance of L0.start L0.end
extrude "Extrude1" add sketch "Sticker" along normal blind 0.01 makes body 1
sketch "Text" plane through (0, 0, 0) normal (0, -1, 0) x (1, 0, 0)
  line L0 (20, 12) -> (0, 12)
  line L1 (0, 12) -> (0, 0)
  line L2 (0, 0) -> (20, 0)
  line L3 (20, 0) -> (20, 12)
  line L4 (0, 0) -> (20, 0) construction
  line L5 (20, 0) -> (20, 12) construction
  line L6 (20, 12) -> (0, 12) construction
  line L7 (0, 12) -> (0, 0) construction
  dimension "d5" = 5
  text T0 "Back" font "Arial" height 5 align centre middle in box 20 x 12 at (0, 0) x (1, 0) y (0, 1) spacing 1 kerned
  constraint coincident L2.end
  constraint coincident L0.end
extrude "Extrude2" add sketch "Text" along normal blind 0.01 separate body text T0 makes body 2 at (14.6982, 0, 5.8829) makes body 3 at (11.2962, 0, 4.2151) makes body 4 at (9.8356, 0, 4.5282) makes body 5 at (2.7257, 0, 5.9363)
equation "d8 = 'Back'"
named bodies: "Sticker", "Text 4", "Text 3", "Text 2", "Text 1"
